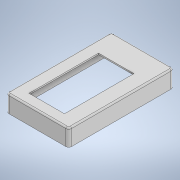
# Autodesk Inventor part: wanne
Saved by Autodesk Inventor 2022 (Build 260153000, 153)
## iProperties
Created: 2022-04-04
Part Number: wanne
Material: Generisch
Document SubType Name: Modeling
Designer: ga76xid
Density: 1 g/cm^3
Appearance: Vorgabe
Author: ga76xid
Autodesk Inventor part; units mm, degrees
ref_plane "YZ Plane" through (0, 0, 0) normal (1, 0, 0) x (0, 1, 0)
ref_plane "XZ Plane" through (0, 0, 0) normal (0, 1, 0) x (-1, 0, 0)
ref_plane "XY Plane" through (0, 0, 0) normal (0, 0, 1) x (1, 0, 0)
sketch "Skizze1" plane through (0, 0, 0) normal (0, 1, 0) x (-1, 0, 0)
  line L0 (1, 0) -> (40, 0)
  line L1 (41, 1) -> (41, 70)
  line L2 (40, 71) -> (1, 71)
  line L3 (0, 70) -> (0, 1)
  line L4 (42.5, 70.5) -> (42.5, 0.5)
  line L5 (40.5, -1.5) -> (0.5, -1.5)
  line L6 (-1.5, 0.5) -> (-1.5, 70.5)
  line L7 (0.5, 72.5) -> (40.5, 72.5)
  arc A0 (42.5, 70.5) -> (40.5, 72.5) centre (40.5, 70.5) ccw
  arc A1 (40.5, -1.5) -> (42.5, 0.5) centre (40.5, 0.5) ccw
  arc A2 (-1.5, 0.5) -> (0.5, -1.5) centre (0.5, 0.5) ccw
  arc A3 (0.5, 72.5) -> (-1.5, 70.5) centre (0.5, 70.5) ccw
  arc A4 (41, 70) -> (40, 71) centre (40, 70) ccw
  arc A5 (40, 0) -> (41, 1) centre (40, 1) ccw
  arc A6 (0, 1) -> (1, 0) centre (1, 1) ccw
  arc A7 (1, 71) -> (0, 70) centre (1, 70) ccw
  point P0 (0, 0)
  point P1 (41, 71)
  point P2 (41, 0)
  point P3 (0, 71)
  dimension "d0" = 41
  dimension "d1" = 71
  dimension "d2" = 1.5
  dimension "d3" = 2
  dimension "d4" = 1
  constraints: 16 end point, 16 point on circle, 16 tangent, 8 centre point, 8 point on line, 6 equal radius, 4 parallel, 2 perpendicular, 1 horizontal, 3 other
  measures "d0" distance of point (0, 71) point (41, 71)
  measures "d1" distance of point (41, 71) point (41, 0)
  measures "d2" distance between parallel lines of L1 L4
  measures "d3" radius of A0
  measures "d4" radius of A4
extrude "Extrusion1" add sketch "Skizze1" along normal blind 11
sketch "Skizze2" plane through (0, 11, 0) normal (0, 1, 0) x (1, 0, 0)
  line L0 (1.5, -70.5) -> (1.5, -0.5) projected
  arc A0 (1.5, -0.5) -> (-0.5, 1.5) centre (-0.5, -0.5) ccw projected
  line L1 (-0.5, 1.5) -> (-40.5, 1.5) projected
  arc A1 (-40.5, 1.5) -> (-42.5, -0.5) centre (-40.5, -0.5) ccw projected
  line L2 (-42.5, -0.5) -> (-42.5, -70.5) projected
  arc A2 (-42.5, -70.5) -> (-40.5, -72.5) centre (-40.5, -70.5) ccw projected
  line L3 (-40.5, -72.5) -> (-0.5, -72.5) projected
  arc A3 (-0.5, -72.5) -> (1.5, -70.5) centre (-0.5, -70.5) ccw projected
  arc A4 (0, -1) -> (-1, 0) centre (-1, -1) ccw projected
  line L4 (0, -1) -> (0, -70) projected
  arc A5 (-1, -71) -> (0, -70) centre (-1, -70) ccw projected
  line L5 (-1, -71) -> (-40, -71) projected
  arc A6 (-41, -70) -> (-40, -71) centre (-40, -70) ccw projected
  line L6 (-41, -70) -> (-41, -1) projected
  arc A7 (-40, 0) -> (-41, -1) centre (-40, -1) ccw projected
  line L7 (-40, 0) -> (-1, 0) projected
  point P0 (0, 0)
extrude "Extrusion2" add sketch "Skizze2" along normal blind 1 contours A3 L3 A2 L2 A1 L1 A0 L0 | L4 A5 L5 A6 L6 A7 L7 A4
fillet "Rundung1" radius 1 8 edges at (0.9142, 12, -0.9142) (-20.5, 12, -1.5) (-41.9142, 12, -0.9142) (-42.5, 12, 35.5) (-41.9142, 12, 71.9142) (-20.5, 12, 72.5) (0.9142, 12, 71.9142) (1.5, 12, 35.5)
sketch "Skizze5" plane through (0, 12, 0) normal (0, 1, 0) x (1, 0, 0)
  line L0 (-34, -65) -> (-9, -65)
  line L1 (-9, -65) -> (-9, -16)
  line L2 (-9, -16) -> (-34, -16)
  line L3 (-34, -16) -> (-34, -65)
  line L4 (-40, 0) -> (-1, 0) projected
  line L5 (-41, -70) -> (-41, -1) projected
  line L6 (0, -1) -> (0, -70) projected
  point P0 (0, 0)
  dimension "d22" = 16
  dimension "d23" = 7
  dimension "d24" = 9
  dimension "d25" = 49
  constraints: 8 end point, 2 parallel, 1 horizontal, 1 perpendicular
  measures "d22" distance between parallel lines of L2 L4
  measures "d23" distance between parallel lines of L5 L3
  measures "d24" distance between parallel lines of L1 L6
  measures "d25" distance between parallel lines of L0 L2
extrude "Extrusion5" cut sketch "Skizze5" against normal blind 10
sketch "Skizze6" plane through (-0.5, 0, -1.5) normal (0, 0, -1) x (-1, 0, 0)
  line L0 (39.5, 0) -> (0.5, 0) projected
  line L1 (25, 0) -> (15, 0)
  line L2 (15, 0) -> (15, 8)
  line L3 (15, 8) -> (25, 8)
  line L4 (25, 8) -> (25, 0)
  line L5 (42, 0) -> (42, 11) projected
  point P0 (-0.5, 0)
  dimension "d28" = 8
  dimension "d29" = 10
  dimension "d30" = 17
  constraints: 8 end point, 2 parallel, 1 horizontal, 1 perpendicular, 1 point on line
  measures "d28" distance between parallel lines of L3 L0
  measures "d29" distance between parallel lines of L2 L4
  measures "d30" distance between parallel lines of L5 L4
extrude "Extrusion6" cut sketch "Skizze6" against normal blind 11
